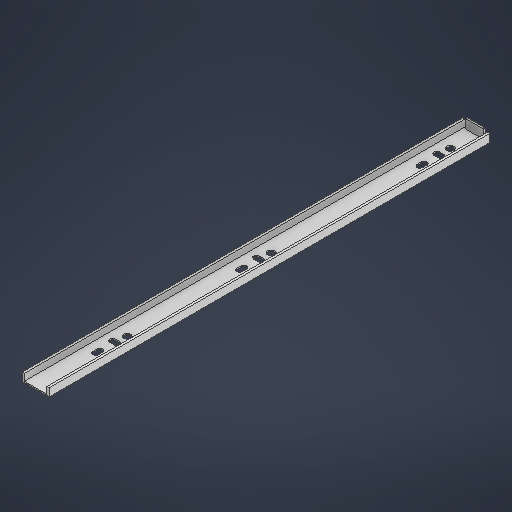
# Autodesk Inventor part: 3 часть направляшки
Saved by Autodesk Inventor 2025 (Build 290162000, 162)
## iProperties
Created: 2024-11-23
Part Number: 3 часть направляшки
Material: Типовые
Document SubType Name: Modeling
Designer: Phantom
Density: 1 g/cm^3
Appearance: По умолчанию
Author: Phantom
Autodesk Inventor part; units mm, degrees
ref_plane "YZ Plane" through (0, 0, 0) normal (1, 0, 0) x (0, 1, 0)
ref_plane "XZ Plane" through (0, 0, 0) normal (0, 1, 0) x (-1, 0, 0)
ref_plane "XY Plane" through (0, 0, 0) normal (0, 0, 1) x (1, 0, 0)
sketch "Эскиз1" plane through (0, 0, 0) normal (0, 0, 1) x (1, 0, 0)
  line L0 (0, 0) -> (24, 0)
  line L1 (24, 0) -> (24, 7)
  line L2 (24, 7) -> (0, 7)
  line L3 (0, 7) -> (0, 0)
  line L4 (0, 1) -> (24, 1)
  line L5 (2, 7) -> (2, 0)
  line L6 (22, 7) -> (22, 0)
  point P0 (0, 3.5)
  point P1 (12, 0)
  point P2 (2, 1)
  point P3 (22, 1)
  dimension "d0" = 24
  dimension "d1" = 7
  dimension "d2" = 2
  dimension "d3" = 2
  dimension "d4" = 1
  constraints: 14 end point, 4 perpendicular, 4 point on line, 2 midpoint, 2 parallel, 1 horizontal
  measures "d0" distance of L2.end L1.end
  measures "d1" distance of L1.end L0.end
  measures "d2" distance from line of point (0, 3.5) L5
  measures "d3" distance between parallel lines of L1 L6
  measures "d4" distance from line of point (12, 0) L4
extrude "Выдавливание1" add sketch "Эскиз1" along normal blind 390 contours L3 L4 L5 L0 | L5 L4 L6 L0 | L3 L2 L5 L4 | L6 L4 L1 L0 | L6 L2 L1 L4
sketch "Эскиз3" plane through (0, 0, 0) normal (0, -1, 0) x (1, 0, 0)
  line L0 (12.0032, 0) -> (12, 390)
  line L1 (22, 390) -> (2, 390) projected
  circle A0 centre (12.003, 23) radius 3.25
  line L2 (0, 0) -> (24, 0) projected
  line L3 (7.5, 33) -> (16.5, 33) construction
  line L4 (24, 0) -> (24, 390) projected
  line L5 (10, 30.5) -> (14, 30.5)
  line L6 (14, 35.5) -> (10, 35.5)
  arc A1 (10, 35.5) -> (10, 30.5) centre (10, 33) ccw
  arc A2 (14, 30.5) -> (14, 35.5) centre (14, 33) ccw
  line L7 (12.0029, 43.5) -> (12.0028, 52.5) construction
  line L8 (14.5028, 46) -> (14.5028, 50)
  line L9 (9.5028, 50) -> (9.5028, 46)
  arc A3 (9.5028, 46) -> (14.5028, 46) centre (12.0028, 46) ccw
  arc A4 (14.5028, 50) -> (9.5028, 50) centre (12.0028, 50) ccw
  circle A5 centre (12.9217, 182.4968) radius 3.25
  line L10 (7.4336, 192.5395) -> (16.4317, 192.3559) construction
  line L11 (9.8821, 189.989) -> (13.8813, 189.9074)
  line L12 (13.9833, 194.9064) -> (9.9841, 194.988)
  arc A6 (9.9841, 194.988) -> (9.8821, 189.989) centre (9.9331, 192.4885) ccw
  arc A7 (13.8813, 189.9074) -> (13.9833, 194.9064) centre (13.9323, 192.4069) ccw
  line L13 (11.9196, 202.9469) -> (11.9271, 211.9469) construction
  line L14 (14.4217, 205.4448) -> (14.425, 209.4448)
  line L15 (9.425, 209.449) -> (9.4217, 205.449)
  arc A8 (9.4217, 205.449) -> (14.4217, 205.4448) centre (11.9217, 205.4469) ccw
  arc A9 (14.425, 209.4448) -> (9.425, 209.449) centre (11.925, 209.4469) ccw
  line L16 (11.9646, 330.3923) -> (11.9626, 339.3923) construction
  line L17 (14.464, 332.8928) -> (14.4632, 336.8928)
  arc A10 (14.4632, 336.8928) -> (9.4632, 336.8918) centre (11.9632, 336.8923) ccw
  arc A11 (9.464, 332.8918) -> (14.464, 332.8928) centre (11.964, 332.8923) ccw
  line L18 (7.4209, 320.0033) -> (16.4182, 319.7828) construction
  arc A12 (9.9814, 322.4413) -> (9.8589, 317.4428) centre (9.9201, 319.9421) ccw
  circle A13 centre (12.9562, 309.9469) radius 3.25
  line L19 (9.4632, 336.8918) -> (9.464, 332.8918)
  line L20 (13.9802, 322.3433) -> (9.9814, 322.4413)
  arc A14 (13.8577, 317.3448) -> (13.9802, 322.3433) centre (13.9189, 319.844) ccw
  line L21 (9.8589, 317.4428) -> (13.8577, 317.3448)
  point P0 (12, 33)
  point P1 (12.0028, 48)
  point P2 (12, 35.5)
  point P3 (11.9327, 192.4477)
  point P4 (11.9233, 207.4469)
  point P5 (11.9837, 194.9472)
  point P6 (12.0028, 52.5)
  point P7 (11.9636, 334.8923)
  point P8 (11.9646, 330.3923)
  point P9 (11.9195, 319.8931)
  point P10 (11.9808, 322.3923)
  point P11 (11.9271, 211.9469)
  dimension "d7" = 6.5
  dimension "d8" = 23
  dimension "d9" = 9
  dimension "d10" = 5
  dimension "d11" = 10
  dimension "d12" = 9
  dimension "d13" = 5
  dimension "d14" = 8
  dimension "d15" = 6.5
  dimension "d16" = 9
  dimension "d17" = 5
  dimension "d18" = 10
  dimension "d19" = 9
  dimension "d20" = 5
  dimension "d21" = 8
  dimension "d22" = 130
  dimension "d23" = 6.5
  dimension "d24" = 9
  dimension "d25" = 5
  dimension "d26" = 10
  dimension "d27" = 9
  dimension "d28" = 5
  dimension "d29" = 8
  dimension "d30" = 98
  constraints: 50 end point, 41 point on circle, 24 tangent, 15 centre point, 15 point on line, 10 midpoint, 6 parallel, 1 perpendicular
  measures "d7" diameter of A0
  measures "d8" distance from line of A0.centre L2
  measures "d9" distance of L3.start L3.end
  measures "d10" diameter of A2
  measures "d11" distance of point (12, 33) A0.centre
  measures "d12" distance of L7.start L7.end
  measures "d13" diameter of A4
  measures "d14" distance of point (12.003, 43.5) point (12, 35.5)
  measures "d15" diameter of A5
  measures "d16" distance of L10.start L10.end
  measures "d17" diameter of A7
  measures "d18" distance of point (11.933, 192.448) A5.centre
  measures "d19" distance of L13.start L13.end
  measures "d20" diameter of A9
  measures "d21" distance of point (11.92, 202.947) point (11.984, 194.947)
  measures "d22" distance of A5.centre point (12.003, 52.5)
  measures "d23" diameter of A13
  measures "d24" distance of L18.start L18.end
  measures "d25" diameter of A14
  measures "d26" distance of point (11.92, 319.893) A13.centre
  measures "d27" distance of L16.start L16.end
  measures "d28" diameter of A10
  measures "d29" distance of point (11.965, 330.392) point (11.981, 322.392)
  measures "d30" vertical distance of point (11.927, 211.947) A13.centre
extrude "Выдавливание2" cut sketch "Эскиз3" against normal blind 10
sketch "Эскиз4" plane through (0, 0, 0) normal (0, 0, -1) x (-1, 0, 0)
  line L0 (-2, 7) -> (0, 7) projected
  line L1 (-2, 1) -> (-2, 7) projected
  line L2 (-22, 1) -> (-2, 1) projected
  line L3 (-22, 7) -> (-22, 1) projected
  line L4 (-24, 7) -> (-22, 7) projected
  line L5 (-24, 0) -> (-24, 7) projected
  line L6 (0, 0) -> (-24, 0) projected
  line L7 (0, 7) -> (0, 0) projected
  line L8 (-12, 9) -> (-20, 9)
  line L9 (-20, 9) -> (-20, 0)
  line L10 (-12, 9) -> (-4, 9)
  line L11 (-4, 9) -> (-4, 0)
  point P0 (-20, 1)
  point P1 (-4, 1)
  constraints: 8 end point, 3 point on line, 2 perpendicular
extrude "Выдавливание3" add sketch "Эскиз4" against normal blind 1.5 contours L2 L9 L8 L10 L11
